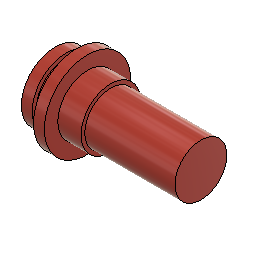
Power Connector (Autodesk Fusion 360 design; units mm, degrees)
Autodesk Fusion 360 part; units mm, degrees
sketch "Sketch1" plane through (0, 0, 0) normal (0, 0, 1) x (1, 0, 0)
  circle A0 centre (0, 0) radius 6.25
  circle A1 centre (0, 0) radius 4.8
  circle A2 centre (0, 0) radius 5.5
  circle A3 centre (0, 0) radius 8
  dimension "d43" = 12.5
  dimension "d44" = 9.6
  dimension "d45" = 11
  dimension "d133" = 16
  dimension "d137" = 0
  dimension "d138" = 0
  dimension "d139" = 0
  dimension "d140" = 0
  constraint coincident A0.centre A1.centre
  constraint concentric A0 A3
  measures "d43" diameter of A0
  measures "d44" diameter of A1
  measures "d45" diameter of A2
  measures "d133" diameter of A3
extrude "Extrude1" add sketch "Sketch1" along normal blind 2 contours A0 | A1 | A2
extrude "Extrude2" add sketch "Sketch1" along normal blind 10.3 contours A1 | A2
extrude "Extrude3" add sketch "Sketch1" along normal blind 27 contours A1
extrude "Extrude4" add sketch "Sketch1" along normal blind 2 from surface at 4 contours A0 | A3
hole "Hole1" at (0, 0, 0) direction (0, 0, 1) diameter 5.64 depth 11 tip angle 180
cylinder "CylinderPrimitive1" add diameter 1.8 height 20 placed x (1, 0, 0) y (0, 1, 0) z (0, 0, 1) at (0, 0, 0)
fillet "Fillet1" radius 0.9 1 edges at (-0.8391, 0.3255, 0)
move_body "Move1" bodies 1 to x (0, 0, -1) y (0, 1, 0) z (1, 0, 0) at (-6.25, 0, -6.25)
named bodies: "Power Connector"
